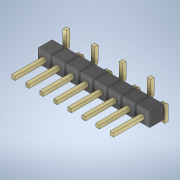
# Autodesk Inventor part: 1x8 SMD Header
Saved by Autodesk Inventor 2020 (Build 240168000, 168)
## iProperties
Created: 2019-12-15
Part Number: 1x8 SMD Header
Material: Generic
Document SubType Name: Modeling
Designer: torto
Density: 1 g/cm^3
Appearance: Smooth - Black
Author: torto
Autodesk Inventor part; units mm, degrees
sketch "Sketch1" plane through (0, 0, 0) normal (0, 0, 1) x (1, 0, 0)
  line L0 (0, 0) -> (2.54, 0)
  line L1 (2.54, 0) -> (2.54, 2.54)
  line L2 (2.54, 2.54) -> (0, 2.54)
  line L3 (0, 2.54) -> (0, 0)
  line L4 (1.27, 2.54) -> (1.27, 0) construction
  line L5 (0, 1.27) -> (2.54, 1.27) construction
  line L6 (0.9525, 1.5875) -> (1.5875, 1.5875)
  line L7 (1.5875, 1.5875) -> (1.5875, 0.9525)
  line L8 (1.5875, 0.9525) -> (0.9525, 0.9525)
  line L9 (0.9525, 0.9525) -> (0.9525, 1.5875)
  line L10 (0.9525, 1.5875) -> (1.5875, 0.9525) construction
  line L11 (1.5875, 1.5875) -> (0.9525, 0.9525) construction
  line L12 (5.08, 2.54) -> (2.54, 2.54)
  line L13 (5.08, 0) -> (5.08, 2.54)
  line L14 (2.54, 0) -> (5.08, 0)
  line L15 (2.54, 2.54) -> (2.54, 0)
  line L16 (3.4925, 0.9525) -> (3.4925, 1.5875)
  line L17 (4.1275, 0.9525) -> (3.4925, 0.9525)
  line L18 (4.1275, 1.5875) -> (4.1275, 0.9525)
  line L19 (3.4925, 1.5875) -> (4.1275, 1.5875)
  line L20 (7.62, 2.54) -> (5.08, 2.54)
  line L21 (7.62, 0) -> (7.62, 2.54)
  line L22 (5.08, 0) -> (7.62, 0)
  line L23 (5.08, 2.54) -> (5.08, 0)
  line L24 (6.0325, 0.9525) -> (6.0325, 1.5875)
  line L25 (6.6675, 0.9525) -> (6.0325, 0.9525)
  line L26 (6.6675, 1.5875) -> (6.6675, 0.9525)
  line L27 (6.0325, 1.5875) -> (6.6675, 1.5875)
  line L28 (10.16, 2.54) -> (7.62, 2.54)
  line L29 (10.16, 0) -> (10.16, 2.54)
  line L30 (7.62, 0) -> (10.16, 0)
  line L31 (7.62, 2.54) -> (7.62, 0)
  line L32 (8.5725, 0.9525) -> (8.5725, 1.5875)
  line L33 (9.2075, 0.9525) -> (8.5725, 0.9525)
  line L34 (9.2075, 1.5875) -> (9.2075, 0.9525)
  line L35 (8.5725, 1.5875) -> (9.2075, 1.5875)
  line L36 (12.7, 2.54) -> (10.16, 2.54)
  line L37 (12.7, 0) -> (12.7, 2.54)
  line L38 (10.16, 0) -> (12.7, 0)
  line L39 (10.16, 2.54) -> (10.16, 0)
  line L40 (11.1125, 0.9525) -> (11.1125, 1.5875)
  line L41 (11.7475, 0.9525) -> (11.1125, 0.9525)
  line L42 (11.7475, 1.5875) -> (11.7475, 0.9525)
  line L43 (11.1125, 1.5875) -> (11.7475, 1.5875)
  line L44 (15.24, 2.54) -> (12.7, 2.54)
  line L45 (15.24, 0) -> (15.24, 2.54)
  line L46 (12.7, 0) -> (15.24, 0)
  line L47 (12.7, 2.54) -> (12.7, 0)
  line L48 (13.6525, 0.9525) -> (13.6525, 1.5875)
  line L49 (14.2875, 0.9525) -> (13.6525, 0.9525)
  line L50 (14.2875, 1.5875) -> (14.2875, 0.9525)
  line L51 (13.6525, 1.5875) -> (14.2875, 1.5875)
  line L52 (17.78, 2.54) -> (15.24, 2.54)
  line L53 (17.78, 0) -> (17.78, 2.54)
  line L54 (15.24, 0) -> (17.78, 0)
  line L55 (15.24, 2.54) -> (15.24, 0)
  line L56 (16.1925, 0.9525) -> (16.1925, 1.5875)
  line L57 (16.8275, 0.9525) -> (16.1925, 0.9525)
  line L58 (16.8275, 1.5875) -> (16.8275, 0.9525)
  line L59 (16.1925, 1.5875) -> (16.8275, 1.5875)
  line L60 (20.32, 2.54) -> (17.78, 2.54)
  line L61 (20.32, 0) -> (20.32, 2.54)
  line L62 (17.78, 0) -> (20.32, 0)
  line L63 (17.78, 2.54) -> (17.78, 0)
  line L64 (18.7325, 0.9525) -> (18.7325, 1.5875)
  line L65 (19.3675, 0.9525) -> (18.7325, 0.9525)
  line L66 (19.3675, 1.5875) -> (19.3675, 0.9525)
  line L67 (18.7325, 1.5875) -> (19.3675, 1.5875)
  line L68 (2.54, 2.54) -> (2.413, 2.54)
  line L69 (2.413, 2.54) -> (2.413, 2.413) construction
  line L70 (2.413, 2.413) -> (2.54, 2.413) construction
  line L71 (2.54, 2.413) -> (2.54, 2.54)
  line L72 (2.413, 2.54) -> (2.54, 2.413)
  line L73 (0.127, 2.54) -> (0.127, 2.413) construction
  line L74 (0.127, 2.413) -> (0, 2.413) construction
  line L75 (0.127, 2.54) -> (0, 2.413)
  line L76 (2.413, 0) -> (2.54, 0.127)
  line L77 (0.127, 0) -> (0, 0.127)
  line L78 (2.667, 2.54) -> (2.54, 2.413)
  line L79 (2.667, 0) -> (2.54, 0.127)
  line L80 (4.953, 0) -> (5.08, 0.127)
  line L81 (4.953, 2.54) -> (5.08, 2.413)
  line L82 (5.207, 2.54) -> (5.08, 2.413)
  line L83 (5.207, 0) -> (5.08, 0.127)
  line L84 (7.493, 0) -> (7.62, 0.127)
  line L85 (7.493, 2.54) -> (7.62, 2.413)
  line L86 (7.747, 2.54) -> (7.62, 2.413)
  line L87 (7.747, 0) -> (7.62, 0.127)
  line L88 (10.033, 0) -> (10.16, 0.127)
  line L89 (10.033, 2.54) -> (10.16, 2.413)
  line L90 (10.287, 2.54) -> (10.16, 2.413)
  line L91 (10.287, 0) -> (10.16, 0.127)
  line L92 (12.573, 0) -> (12.7, 0.127)
  line L93 (12.573, 2.54) -> (12.7, 2.413)
  line L94 (12.827, 2.54) -> (12.7, 2.413)
  line L95 (12.827, 0) -> (12.7, 0.127)
  line L96 (15.113, 0) -> (15.24, 0.127)
  line L97 (15.113, 2.54) -> (15.24, 2.413)
  line L98 (15.367, 2.54) -> (15.24, 2.413)
  line L99 (15.367, 0) -> (15.24, 0.127)
  line L100 (17.653, 0) -> (17.78, 0.127)
  line L101 (17.653, 2.54) -> (17.78, 2.413)
  line L102 (17.907, 2.54) -> (17.78, 2.413)
  line L103 (17.907, 0) -> (17.78, 0.127)
  line L104 (20.193, 0) -> (20.32, 0.127)
  line L105 (20.193, 2.54) -> (20.32, 2.413)
  point P0 (1.27, 1.27)
  point P1 (3.81, 2.54)
  point P2 (5.08, 1.27)
  point P3 (3.81, 0)
  point P4 (6.35, 2.54)
  point P5 (7.62, 1.27)
  point P6 (6.35, 0)
  point P7 (5.08, 1.27)
  point P8 (8.89, 2.54)
  point P9 (10.16, 1.27)
  point P10 (8.89, 0)
  point P11 (7.62, 1.27)
  point P12 (11.43, 2.54)
  point P13 (12.7, 1.27)
  point P14 (11.43, 0)
  point P15 (10.16, 1.27)
  point P16 (13.97, 2.54)
  point P17 (15.24, 1.27)
  point P18 (13.97, 0)
  point P19 (12.7, 1.27)
  point P20 (16.51, 2.54)
  point P21 (17.78, 1.27)
  point P22 (16.51, 0)
  point P23 (15.24, 1.27)
  point P24 (19.05, 2.54)
  point P25 (20.32, 1.27)
  point P26 (19.05, 0)
  point P27 (17.78, 1.27)
  dimension "d1" = 2.54
  dimension "d2" = 2.54
  dimension "PinThickness" = 0.635
  dimension "d4" = 0.635
  dimension "d7" = 2.54
  dimension "CasingChamfer" = 0.127
  dimension "d15" = 0.127
  dimension "d18" = 2.54
  constraints: 212 end point, 7 midpoint, 7 symmetric about line, 6 parallel, 5 horizontal, 3 perpendicular, 1 collinear, 223 other
  measures "d1" distance of L0.end L1.end
  measures "d2" distance of L1.end L2.end
  measures "PinThickness" distance of L7.end L8.end
  measures "d4" distance of L6.end L7.end
  measures "d7" distance of L1.end L12.start
  measures "CasingChamfer" distance of L70.end L69.end
  measures "d15" distance of L68.end L69.end
  measures "d18" distance of L73.start L78.start
extrude "Extrusion2" add sketch "Sketch1" along normal blind 2.54 contours L77 L3 L75 L2 L72 L1 L76 L0 | L1 L78 L12 L81 L13 L80 L14 L79 | L13 L82 L20 L85 L21 L84 L22 L83 | L21 L86 L28 L89 L29 L88 L30 L87 | L29 L90 L36 L93 L37 L92 L38 L91 | L37 L94 L44 L97 L45 L96 L46 L95 | L45 L98 L52 L101 L53 L100 L54 L99 | L53 L102 L60 L105 L61 L104 L62 L103
sketch "Sketch4" plane through (0.127, 0, 0) normal (0, -1, 0) x (1, 0, 0)
  line L0 (2.413, 2.54) -> (2.286, 2.54) projected
  line L1 (2.286, 2.54) -> (2.413, 2.54)
  line L2 (2.413, 2.54) -> (2.413, 2.413)
  line L3 (2.413, 0) -> (2.413, 2.54) projected
  line L4 (2.413, 2.413) -> (2.286, 2.54)
  point P0 (-0.127, 0)
  dimension "d27" = 0.127
  constraints: 6 end point, 1 collinear, 1 point on line
  measures "d27" distance of L0.start L2.end
extrude "Extrusion3" cut sketch "Sketch4" against normal blind 2.54
ref_plane "Work Plane1" through (1.27, 1.5875, 2.54) normal (1, 0, 0) x (0, 1, 0)
mirror "Mirror1" about plane through (1.27, 1.5875, 2.54) normal (1, 0, 0) of "Extrusion3"
sketch "Sketch6" plane through (0, 0.127, 0) normal (-1, 0, 0) x (0, 0, 1)
  line L0 (2.413, 2.286) -> (2.54, 2.413) projected
  line L1 (2.413, 0) -> (2.413, 2.286) projected
  line L2 (2.54, 2.413) -> (2.413, 2.413)
  line L3 (2.413, 2.413) -> (2.413, 2.286)
  line L4 (2.413, 2.286) -> (2.54, 2.286)
  line L5 (2.54, 2.286) -> (2.54, 2.413)
  line L6 (2.413, 2.413) -> (2.54, 2.286)
  point P0 (0, -0.127)
  constraints: 10 end point, 2 parallel, 1 horizontal, 1 perpendicular
extrude "Extrusion5" cut sketch "Sketch6" against normal blind 2.54 contours L6 L2 L0 | L0 L5 L6
ref_plane "Work Plane3" through (0.9525, 1.27, 2.54) normal (0, -1, 0) x (1, 0, 0)
mirror "Mirror2" about plane through (0.9525, 1.27, 2.54) normal (0, -1, 0) of "Extrusion5"
pattern_linear "Rectangular Pattern1" count 8 spacing 2.54 along (1, 0, 0) of "Extrusion3", "Mirror1"
pattern_linear "Rectangular Pattern2" count 8 spacing 2.54 along (1, 0, 0) of "Extrusion5", "Mirror2"
ref_plane "Work Plane5" through (0.127, 0, 1.2065) normal (0, 0, 1) x (1, 0, 0)
mirror "Mirror4" about plane through (0.127, 0, 1.2065) normal (0, 0, 1)
sketch "Sketch7" plane through (0, 0, 2.54) normal (0, 0, 1) x (1, 0, 0)
  line L0 (0.9525, 0.9525) -> (0.9525, 1.5875) projected
  line L1 (1.5875, 1.5875) -> (1.5875, 0.9525) projected
  line L2 (0.9525, 1.5875) -> (1.5875, 1.5875)
  line L3 (1.5875, 1.5875) -> (1.5875, 0.9525)
  line L4 (1.5875, 0.9525) -> (0.9525, 0.9525)
  line L5 (0.9525, 0.9525) -> (0.9525, 1.5875)
  point P0 (0, 0)
  constraints: 8 end point, 2 parallel, 1 horizontal, 1 perpendicular
extrude "Extrusion6" add sketch "Sketch7" along normal blind 5.588
pattern_linear "Rectangular Pattern3" count 8 spacing 2.54 along (1, 0, 0) of "Extrusion6"
sketch "Sketch8" plane through (19.3675, 0.9525, 2.54) normal (0, 0, -1) x (-1, 0, 0)
  line L0 (0, 0.635) -> (0, 0) projected
  line L1 (0, 0) -> (0.635, 0) projected
  line L2 (0, 0.635) -> (0.635, 0.635)
  line L3 (0.635, 0.635) -> (0.635, 0)
  line L4 (0.635, 0) -> (0, 0)
  line L5 (0, 0) -> (0, 0.635)
  point P0 (19.3675, -0.9525)
  constraints: 8 end point, 2 parallel, 1 horizontal, 1 perpendicular
extrude "Extrusion8" add sketch "Sketch8" along normal blind 4.318
pattern_linear "Rectangular Pattern4" count 8 spacing 2.54 along (-1, 0, 0) of "Extrusion8"
sketch "Sketch9" plane through (0.9525, 0.9525, -0.127) normal (0, -1, 0) x (1, 0, 0)
  line L0 (0.635, -1.651) -> (0, -1.651) projected
  line L1 (0, -1.651) -> (0.635, -1.651)
  line L2 (0.635, -1.651) -> (0.635, -1.016)
  line L3 (0.635, -1.016) -> (0, -1.016)
  line L4 (0, -1.016) -> (0, -1.651)
  point P0 (-0.9525, 0.127)
  dimension "d54" = 0.635
  dimension "d55" = 0.635
  constraints: 8 end point, 2 parallel, 1 horizontal, 1 perpendicular
  measures "d54" distance of L3.end L2.end
  measures "d55" distance of L2.end L1.end
extrude "Extrusion9" add sketch "Sketch9" against normal blind 3.1115
sketch "Sketch10" plane through (0.9525, 0.9525, -0.127) normal (-1, 0, 0) x (0, 0, 1)
  line L0 (-1.651, 0) -> (-1.651, 0.635) projected
  line L1 (-1.651, 0.635) -> (-1.016, 0.635)
  line L2 (-1.016, 0.635) -> (-1.016, 0)
  line L3 (-1.016, 0) -> (-1.651, 0)
  line L4 (-1.651, 0) -> (-1.651, 0.635)
  arc A0 (-1.651, 0.635) -> (-1.016, 0) centre (-1.016, 0.635) ccw
  point P0 (0.127, -0.9525)
  dimension "d58" = 0.635
  dimension "d59" = 0.635
  dimension "d76" = 0.635
  constraints: 8 end point, 2 parallel, 2 point on circle, 1 centre point, 1 horizontal, 1 perpendicular
  measures "d58" distance of L2.end L3.end
  measures "d59" distance of L1.end L2.end
  measures "d76" radius of A0
extrude "Extrusion10" cut sketch "Sketch10" against normal blind 0.635 contours L0 A0 L3
pattern_linear "Rectangular Pattern5" count 4 spacing 5.08 along (1, 0, 0) of "Extrusion9", "Extrusion10"
sketch "Sketch12" plane through (3.4925, 1.5875, -0.127) normal (0, 1, 0) x (1, 0, 0)
  line L0 (0, 0) -> (0, 1.651) projected
  line L1 (0, 1.651) -> (0.635, 1.651)
  line L2 (0.635, 1.651) -> (0.635, 1.016)
  line L3 (0.635, 1.016) -> (0, 1.016)
  line L4 (0, 1.016) -> (0, 1.651)
  point P0 (-3.4925, -0.127)
  dimension "d66" = 0.635
  dimension "d67" = 0.635
  constraints: 8 end point, 2 parallel, 1 horizontal, 1 perpendicular
  measures "d66" distance of L2.end L3.end
  measures "d67" distance of L1.end L2.end
extrude "Extrusion11" add sketch "Sketch12" against normal blind 3.1115
sketch "Sketch14" plane through (3.4925, 0.9525, -0.127) normal (-1, 0, 0) x (0, 0, 1)
  line L0 (0, 0) -> (-1.016, 0) projected
  line L1 (-1.016, 0) -> (-1.016, -2.4765) projected
  line L2 (0, 0.635) -> (-1.651, 0.635) projected
  line L3 (-1.651, 0.635) -> (-1.016, 0.635)
  line L4 (-1.016, 0.635) -> (-1.016, 0)
  line L5 (-1.016, 0) -> (-1.651, 0)
  line L6 (-1.651, 0) -> (-1.651, 0.635)
  arc A0 (-1.016, 0.635) -> (-1.651, 0) centre (-1.016, 0) ccw
  point P0 (0.127, -0.9525)
  point P1 (-1.016, 3.1115)
  dimension "d78" = 0.635
  constraints: 8 end point, 2 parallel, 2 point on circle, 1 centre point, 1 horizontal, 1 perpendicular
  measures "d78" radius of A0
extrude "Extrusion12" cut sketch "Sketch14" against normal blind 0.635 contours A0 L6 L2
pattern_linear "Rectangular Pattern7" count 4 spacing 5.08 along (1, 0, 0) of "Extrusion11", "Extrusion12"
equation "\"d1\" = StdSpacing"
equation "\"d2\" = StdSpacing"
equation "\"d4\" = PinThickness"
equation "\"d15\" = CasingChamfer"
equation "\"d18\" = StdSpacing"
equation "\"d23\" = StdSpacing"
equation "\"d27\" = CasingChamfer"
equation "\"d28\" = StdSpacing"
equation "\"d34\" = StdSpacing"
equation "\"d38\" = StdSpacing"
equation "\"d41\" = StdSpacing"
equation "\"d46\" = StdSpacing"
equation "\"d53\" = StdSpacing"
equation "\"d54\" = PinThickness"
equation "\"d55\" = PinThickness"
equation "\"d58\" = PinThickness"
equation "\"d59\" = PinThickness"
equation "\"d76\" = PinThickness"
equation "\"d61\" = PinThickness"
equation "\"d65\" = 2 * StdSpacing"
equation "\"d66\" = PinThickness"
equation "\"d67\" = PinThickness"
equation "\"d78\" = PinThickness"
equation "\"d71\" = PinThickness"
equation "\"d81\" = 2 * StdSpacing"
equation "\"StdSpacing\" = 2.54"
body "Solid2"
